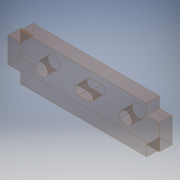
# Autodesk Inventor part: Laser Mount Plate
Saved by Autodesk Inventor 2017 (Build 210142000, 142)
## iProperties
Created: 2017-05-18
Part Number: Laser Mount Plate
Material: Polycarbonate, Smoke
Document SubType Name: Modeling
Designer: yella
Density: 1.2 g/cm^3
Appearance: Polycarbonate - Smoked
Author: yella
Autodesk Inventor part; units mm, degrees
ref_plane "YZ Plane" through (0, 0, 0) normal (1, 0, 0) x (0, 1, 0)
ref_plane "XZ Plane" through (0, 0, 0) normal (0, 1, 0) x (-1, 0, 0)
ref_plane "XY Plane" through (0, 0, 0) normal (0, 0, 1) x (1, 0, 0)
sketch "Sketch1" plane through (0, 0, 0) normal (0, 1, 0) x (-1, 0, 0)
  line L0 (0, 0) -> (0, -3)
  line L1 (0, -3) -> (3, -3)
  line L2 (3, -3) -> (3, -5.5)
  line L3 (3, -5.5) -> (33, -5.5)
  line L4 (33, -5.5) -> (33, -3)
  line L5 (33, -3) -> (36, -3)
  line L6 (36, -3) -> (36, 3)
  line L7 (36, 3) -> (33, 3)
  line L8 (33, 3) -> (33, 5.5)
  line L9 (33, 5.5) -> (3, 5.5)
  line L10 (3, 5.5) -> (3, 3)
  line L11 (3, 3) -> (0, 3)
  line L12 (0, 3) -> (0, 0)
  circle A0 centre (28, 0) radius 1.5
  line L13 (0, 0) -> (8, 0)
  circle A1 centre (8, 0) radius 1.5
  arc A2 (19.25, -1) -> (19.25, 1) centre (19.25, 0) ccw
  arc A3 (16.75, 1) -> (16.75, -1) centre (16.75, 0) ccw
  line L14 (19.25, 1) -> (16.75, 1)
  line L15 (16.75, -1) -> (19.25, -1)
  dimension "d15" = 3
  dimension "d16" = 3
  dimension "d17" = 2.5
  dimension "d18" = 30
  dimension "d19" = 3
  dimension "d20" = 6
  dimension "d21" = 2.5
  dimension "d22" = 30
  dimension "d26" = 8
  dimension "d27" = 3
  dimension "d31" = 8
  dimension "d34" = 1
  dimension "d35" = 11
  constraints: 32 end point, 9 perpendicular, 4 centre point, 4 point on circle, 4 point on line, 2 horizontal, 2 vertical, 1 coincident, 1 parallel
  measures "d15" distance of L0.start L0.end
  measures "d16" distance of L0.end L1.end
  measures "d17" distance of L1.end L2.end
  measures "d18" distance of L2.end L3.end
  measures "d19" distance of L4.end L5.end
  measures "d20" distance of L5.end L6.end
  measures "d21" distance of L7.end L8.end
  measures "d22" distance of L8.end L9.end
  measures "d26" distance of L0.start L13.end
  measures "d27" diameter of A1
  measures "d31" distance from line of L6 A0.centre
  measures "d34" radius of A2
  measures "d35" distance between parallel lines of L3 L9
extrude "Extrusion1" add sketch "Sketch1" along normal blind 3
body "Solid1"
